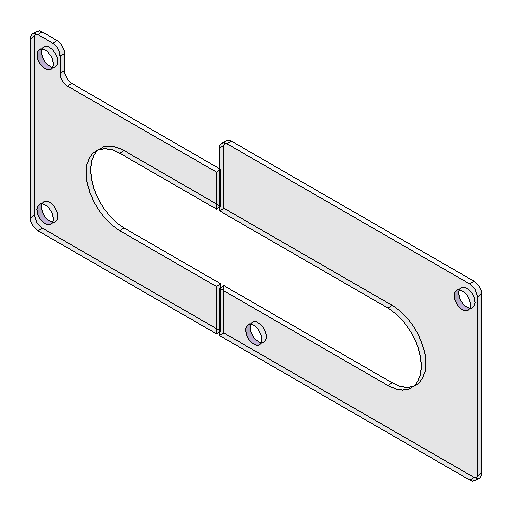
# Autodesk Inventor part: TL20240701-10120CV-012
Saved by Autodesk Inventor 2022.5 (Build 265521000, 521)
## iProperties
Category: FOLLOWER UNIT ASSY
Company: 현대 트랜시스(대유)
Created: 2023-09-30
Part Number: TL20240701-10120CV-012
Project: SW PJT
Checked By: 김형민
Engr Approved By: 김시현
User Status: 2 x18
Material: PC
Description: 0
Document SubType Name: Modeling
Mfg Approved By: 호상태
Designer: 김재훈
Stock Number: 012
Density: 0.357273 g/cm^3
Appearance: Transparency
DETAIL: Coveryor Assembly
M/C TITLE: CJ 제일제당 협동로봇 포장시스탬 PILOT 장비
PARTS NAME: Bracket
SPECIFICATION: TA20221101-CV200000-015
DocNumber: 221118_Standard_v1
Folder: .\
VDS_Category: 엔지니어링
Detail Description: Processed products
Title: PC COVER
Subject: SW차종 시트조립라인
Author: 김재훈
Revision Number: A
Autodesk Inventor part; units mm, degrees
ref_plane "YZ Plane" through (0, 0, 0) normal (1, 0, 0) x (0, 1, 0)
ref_plane "XZ Plane" through (0, 0, 0) normal (0, 1, 0) x (-1, 0, 0)
ref_plane "XY Plane" through (0, 0, 0) normal (0, 0, 1) x (1, 0, 0)
sketch "스케치9" plane through (0, 0, 0) normal (0, 0, 1) x (1, 0, 0)
  line L0 (-150, -57) -> (150, -57)
  line L1 (150, -57) -> (150, 57)
  line L2 (150, 57) -> (-150, 57)
  line L3 (-150, 57) -> (-150, -57)
  line L4 (-150, -57) -> (150, 57) construction
  line L5 (150, -57) -> (-150, 57) construction
  line L6 (93.3891, 57) -> (73.3891, 57) projected
  line L7 (93.3891, -57) -> (93.3891, 15) projected
  point P0 (0, 0)
  point P1 (0, 0)
  dimension "d44" = 114
  dimension "d58" = 300
  constraints: 12 end point, 3 midpoint, 2 parallel, 1 horizontal, 1 perpendicular
  measures "d44" distance of L0.end L1.end
  measures "d58" distance of L0.start L0.end
extrude "돌출4" add sketch "스케치9" along normal mid plane 3
fillet "모깎기2" radius 5 4 edges at (150, 57, 0) (150, -57, 0) (-150, 57, 0) (-150, -57, 0)
sketch "스케치10" plane through (0, 0, 1.5) normal (0, 0, 1) x (1, 0, 0)
  line L0 (150, -52) -> (150, 52) projected
  line L1 (145, 57) -> (-150, 57) projected
  line L2 (-150, -57) -> (145, -57) projected
  line L3 (-150, 52) -> (-150, -52) projected
  point P0 (0, 0)
  point P1 (140, 45)
  point P2 (0, -45)
  point P3 (-140, 45)
  point P4 (-140, -45)
  dimension "d53" = 10
  dimension "d54" = 12
  dimension "d55" = 12
  dimension "d56" = 150
  dimension "d59" = 10
  dimension "d60" = 12
  dimension "d61" = 10
  dimension "d62" = 12
  measures "d53" distance from line of L0 point (140, 45)
  measures "d54" distance from line of L1 point (140, 45)
  measures "d55" distance from line of L2 point (0, -45)
  measures "d56" distance from line of L0 point (0, -45)
  measures "d59" distance from line of L3 point (-140, 45)
  measures "d60" distance from line of L1 point (-140, 45)
  measures "d61" distance from line of L3 point (-140, -45)
  measures "d62" distance from line of L2 point (-140, -45)
hole "구멍3" at (140, 45, 1.5) at (0, -45, 1.5) at (-140, 45, 1.5) at (-140, -45, 1.5) direction (0, 0, -1) diameter 11 end through all clearance for "Socket Head Cap Screw" size "M10" standard "TS Profile"
sketch "스케치11" plane through (0, 0, 1.5) normal (0, 0, 1) x (1, 0, 0)
  line L0 (-25, 57) -> (-23, 57)
  line L1 (-23, 57) -> (-23, -57)
  line L2 (-23, -57) -> (-25, -57)
  line L3 (-25, -57) -> (-25, 57)
  line L4 (150, -52) -> (150, 52) projected
  line L5 (-150, 52) -> (-150, -52) projected
  line L6 (145, 57) -> (-145, 57) projected
  line L7 (-145, -57) -> (145, -57) projected
  line L8 (-90, -7) -> (90, -7) construction
  line L9 (-90, -29.5) -> (90, -29.5)
  line L10 (90, 15.5) -> (-90, 15.5)
  arc A0 (-90, 15.5) -> (-90, -29.5) centre (-90, -7) ccw
  arc A1 (90, -29.5) -> (90, 15.5) centre (90, -7) ccw
  line L11 (-23, 57) -> (-23, 37)
  line L12 (-23, 37) -> (-130, 37)
  line L13 (-130, 37) -> (-130, 57)
  line L14 (-145, 57) -> (145, 57) projected
  line L15 (145, -57) -> (-145, -57) projected
  point P0 (0, 0)
  point P1 (0, -7)
  point P2 (-25, -29.5)
  point P3 (-23, -29.5)
  point P4 (-23, 15.5)
  point P5 (-25, 15.5)
  point P6 (-25, 37)
  point P7 (-25, 57)
  point P8 (-23, 37)
  point P9 (-23, 57)
  dimension "d81" = 300
  dimension "d82" = 20
  dimension "d83" = 107
  dimension "d84" = 20
  dimension "d85" = 2
  dimension "d86" = 173
  dimension "d93" = 64
  dimension "d94" = 45
  dimension "d95" = 150
  dimension "d96" = 180
  constraints: 22 end point, 4 point on circle, 4 point on line, 4 tangent, 3 parallel, 3 perpendicular, 2 centre point, 2 horizontal, 1 midpoint, 1 vertical
  measures "d81" distance between parallel lines of L5 L4
  measures "d82" distance between parallel lines of L13 L5
  measures "d83" distance between parallel lines of L11 L13
  measures "d84" distance between parallel lines of L6 L12
  measures "d85" distance between parallel lines of L11 L3
  measures "d86" distance between parallel lines of L4 L1
  measures "d93" distance between parallel lines of L8 L14
  measures "d94" distance between parallel lines of L9 L10
  measures "d95" distance from line of point (0, -7) L4
  measures "d96" distance of L8.start L8.end
extrude "돌출5" cut sketch "스케치11" against normal through all
fillet "모깎기3" radius 5 3 edges at (-130, 37, 0) (-130, 57, 0) (-23, 57, 0)
